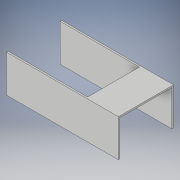
# Autodesk Inventor part: Gen2Plate
Saved by Autodesk Inventor 2017 (Build 210142000, 142)
## iProperties
Created: 2017-12-02
Part Number: Gen2Plate
Material: Generic
Document SubType Name: Modeling
Designer: User
Density: 1 g/cm^3
Appearance: Default
Author: User
Autodesk Inventor part; units mm, degrees
ref_plane "YZ Plane" through (0, 0, 0) normal (1, 0, 0) x (0, 1, 0)
ref_plane "XZ Plane" through (0, 0, 0) normal (0, 1, 0) x (-1, 0, 0)
ref_plane "XY Plane" through (0, 0, 0) normal (0, 0, 1) x (1, 0, 0)
sketch "Sketch1" plane through (0, 0, 0) normal (0, 0, 1) x (1, 0, 0)
  line L0 (0, 0) -> (95.25, 0)
  line L1 (95.25, 0) -> (95.25, -146.05)
  line L2 (95.25, -146.05) -> (0, -146.05)
  line L3 (0, -146.05) -> (0, 0)
  dimension "d0" = 95.25
  dimension "d1" = 146.05
  constraints: 8 end point, 2 parallel, 1 horizontal, 1 perpendicular
  measures "d0" distance of L1.end L2.end
  measures "d1" distance of L0.end L1.end
extrude "Extrusion1" add sketch "Sketch1" along normal blind 6.35
sketch "Sketch2" plane through (0, 0, 6.35) normal (0, 0, 1) x (1, 0, 0)
  line L0 (95.25, 0) -> (0, 0) projected
  line L1 (95.25, 0) -> (-31.75, 0)
  line L2 (-31.75, 0) -> (-31.75, -6.35)
  line L3 (-31.75, -6.35) -> (95.25, -6.35)
  line L4 (95.25, -146.05) -> (95.25, 0) projected
  line L5 (95.25, -6.35) -> (95.25, 0)
  dimension "d4" = 127
  dimension "d5" = 6.35
  constraints: 8 end point, 1 horizontal, 1 parallel, 1 perpendicular, 1 vertical
  measures "d4" distance of L0.start L1.end
  measures "d5" distance of L1.end L2.end
extrude "Extrusion2" add sketch "Sketch2" along normal blind 203.2
sketch "Sketch3" plane through (0, 0, 209.55) normal (0, 0, 1) x (1, 0, 0)
  line L0 (0, 0) -> (95.25, 0) projected
  line L1 (95.25, -146.05) -> (95.25, -6.35) projected
  line L2 (0, 0) -> (95.25, 0)
  line L3 (95.25, 0) -> (95.25, -6.35)
  line L4 (95.25, -6.35) -> (0, -6.35)
  line L5 (0, -6.35) -> (0, 0)
  constraints: 8 end point, 2 parallel, 1 horizontal, 1 perpendicular
extrude "Extrusion3" add sketch "Sketch3" along normal blind 6.35
sketch "Sketch4" plane through (-31.75, -6.35, 6.35) normal (0, -1, 0) x (1, 0, 0)
  line L0 (0, 203.2) -> (31.75, 203.2) projected
  line L1 (31.75, 209.55) -> (127, 209.55) projected
  line L2 (31.75, 203.2) -> (127, 203.2)
  line L3 (127, 203.2) -> (127, 209.55)
  line L4 (127, 209.55) -> (31.75, 209.55)
  line L5 (31.75, 209.55) -> (31.75, 203.2)
  point P0 (31.75, -6.35)
  constraints: 8 end point, 2 parallel, 1 horizontal, 1 perpendicular
extrude "Extrusion4" add sketch "Sketch4" along normal blind 139.7
sketch "Sketch5" plane through (0, -146.05, 0) normal (-1, 0, 0) x (0, 0, 1)
  line L0 (0, 146.05) -> (215.9, 146.05) projected
  line L1 (0, 0) -> (6.35, 0) projected
  line L2 (0, 146.05) -> (6.35, 146.05)
  line L3 (6.35, 146.05) -> (6.35, 0)
  line L4 (6.35, 0) -> (0, 0)
  line L5 (0, 0) -> (0, 146.05)
  constraints: 8 end point, 2 parallel, 1 horizontal, 1 perpendicular
extrude "Extrusion5" add sketch "Sketch5" along normal blind 342.9
sketch "Sketch6" plane through (0, 0, 209.55) normal (-1, 0, 0) x (0, 0, 1)
  line L0 (-209.55, 0) -> (6.35, 0) projected
  line L1 (0, -6.35) -> (0, -146.05) projected
  line L2 (6.35, 0) -> (0, 0)
  line L3 (0, 0) -> (0, -146.05)
  line L4 (0, -146.05) -> (6.35, -146.05)
  line L5 (6.35, -146.05) -> (6.35, 0)
  constraints: 8 end point, 2 parallel, 1 horizontal, 1 perpendicular
extrude "Extrusion6" add sketch "Sketch6" along normal blind 342.9
body "Solid1"
